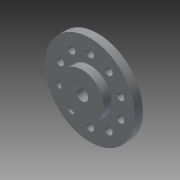
# Autodesk Inventor part: CircularPattern
Saved by Autodesk Inventor 2015 (Build 190159000, 159)
## iProperties
Created: 2017-12-12
Part Number: CircularPattern
Material: Generic
Document SubType Name: Modeling
Designer: Administrator
Density: 1 g/cm^3
Appearance: Default
Author: Administrator
Autodesk Inventor part; units mm, degrees
ref_plane "YZ Plane" through (0, 0, 0) normal (1, 0, 0) x (0, 1, 0)
ref_plane "XZ Plane" through (0, 0, 0) normal (0, 1, 0) x (-1, 0, 0)
ref_plane "XY Plane" through (0, 0, 0) normal (0, 0, 1) x (1, 0, 0)
sketch "Sketch1" plane through (0, 0, 0) normal (0, 0, 1) x (1, 0, 0)
  line L0 (0, 0) -> (0, 25.4)
  line L1 (0, 25.4) -> (12.7, 25.4)
  line L2 (12.7, 25.4) -> (12.7, 63.5)
  line L3 (12.7, 63.5) -> (25.4, 63.5)
  line L4 (25.4, 63.5) -> (25.4, 0)
  line L5 (25.4, 0) -> (0, 0)
  line L6 (0, -9.525) -> (25.4, -9.525)
  dimension "d0" = 25.4
  dimension "d1" = 63.5
  dimension "d2" = 12.7
  dimension "d3" = 25.4
  dimension "d4" = 9.525
  constraints: 14 end point, 5 perpendicular, 1 horizontal, 1 vertical
  measures "d0" distance of L0.start L0.end
  measures "d1" vertical distance of L0.start L2.end
  measures "d2" distance of L2.end L3.end
  measures "d3" distance of L4.end L0.start
  measures "d4" distance between parallel lines of L6 L5
revolve "Revolution1" add sketch "Sketch1" angle 360 about axis through (0, -9.525, 0) along (1, 0, 0)
sketch "Sketch2" plane through (12.7, -9.525, 0) normal (-1, 0, 0) x (0, 0, 1)
  circle A0 centre (0, 0) radius 51.435 construction
  circle A1 centre (0, 0) radius 9.525 projected
  circle A2 centre (0, 0) radius 73.025 projected
  circle A3 centre (0, 0) radius 34.925 projected
  point P0 (0, 9.525)
  point P1 (0, 51.435)
  point P2 (-30.2327, 41.6118)
  point P3 (-48.9176, 15.8943)
  point P4 (-48.9176, -15.8943)
  point P5 (-30.2327, -41.6118)
  point P6 (0, -51.435)
  point P7 (30.2327, -41.6118)
  point P8 (48.9176, -15.8943)
  point P9 (48.9176, 15.8943)
  point P10 (30.2327, 41.6118)
  dimension "d7" = 41.91
  dimension "d17" = 360
  constraints: 2 vertical alignment, 13 other
hole "Hole1" at (12.7, 41.91, 0) direction (1, 0, 0) diameter 12.7 end through all
hole "Hole2" at (12.7, 32.0868, -30.2327) at (12.7, 6.3693, -48.9176) at (12.7, -25.4193, -48.9176) at (12.7, -51.1368, -30.2327) at (12.7, -60.96, 0) at (12.7, -51.1368, 30.2327) at (12.7, -25.4193, 48.9176) at (12.7, 6.3693, 48.9176) at (12.7, 32.0868, 30.2327) direction (1, 0, 0) diameter 12.7 end through all
sketch "Sketch3" plane through (0, -9.525, 0) normal (-1, 0, 0) x (0, 0, 1)
  line L0 (-1.5875, 12.2962) -> (1.5875, 12.2962)
  line L1 (1.5875, 12.2962) -> (1.5875, 9.1212)
  line L2 (1.5875, 9.1212) -> (-1.5875, 9.1212)
  line L3 (-1.5875, 9.1212) -> (-1.5875, 12.2962)
  circle A0 centre (48.9176, 15.8943) radius 6.35 projected
  circle A1 centre (0, 51.435) radius 6.35 projected
  point P0 (0, 9.525)
  point P1 (0, 9.1212)
  point P2 (0, 12.2759)
  dimension "d26" = 3.175
  dimension "d27" = 3.175
  dimension "d29" = 1.5875
  dimension "d30" = 48.9176
  dimension "d31" = 0
  dimension "d33" = 42.3138
  dimension "d34" = 0
  constraints: 8 end point, 2 parallel, 1 horizontal, 1 perpendicular
  measures "d26" distance of L2.end L0.start
  measures "d27" distance of L0.start L0.end
  measures "d29" distance from line of L1 point (0, 12.276)
  measures "d30" horizontal distance of A0.centre point (0, 9.121)
  measures "d31" horizontal distance of point (0, 9.121) point (0, 12.276)
  measures "d33" distance of A1.centre point (0, 9.121)
  measures "d34" distance from line of point (0, 9.121) L2
extrude "Extrusion1" cut sketch "Sketch3" against normal blind 50.8 contours L0 L1 L2 L3
body "Solid1"
